Autodesk Inventor part; units mm, degrees
(part 2 of 2)
sketch "Esquisse17" plane through (0, 1.2, 0) normal (0, 1, 0) x (1, 0, 0)
  line L0 (-1.4817, 5.2601) -> (-1.4817, 7.5121) construction
  line L1 (-1.4817, 7.5121) -> (-0.4817, 7.5121) construction
  line L2 (-0.4817, 7.5121) -> (-0.4817, 5.2601) construction
  line L3 (-0.4817, 5.2601) -> (-1.4817, 5.2601) construction
  line L4 (-1.4819, 10.1681) -> (-1.4819, 12.4202) construction
  line L5 (-1.4819, 12.4202) -> (-0.4819, 12.4202) construction
  line L6 (-0.4819, 12.4202) -> (-0.4819, 10.1681) construction
  line L7 (-0.4819, 10.1681) -> (-1.4819, 10.1681) construction
  line L8 (-1.5006, 15.4095) -> (-1.5006, 17.6616) construction
  line L9 (-1.5006, 17.6616) -> (-0.5006, 17.6616) construction
  line L10 (-0.5006, 17.6616) -> (-0.5006, 15.4095) construction
  line L11 (-0.5006, 15.4095) -> (-1.5006, 15.4095) construction
  line L12 (-4.5935, 7.6677) -> (-4.5935, 9.9198) construction
  line L13 (-4.5935, 9.9198) -> (-3.5935, 9.9198) construction
  line L14 (-3.5935, 9.9198) -> (-3.5935, 7.6677) construction
  line L15 (-3.5935, 7.6677) -> (-4.5935, 7.6677) construction
  line L16 (-3.5936, 12.8721) -> (-4.5936, 12.8721) construction
  line L17 (-4.5936, 12.8721) -> (-4.5936, 15.1241) construction
  line L18 (-4.5936, 15.1241) -> (-3.5936, 15.1241) construction
  line L19 (-3.5936, 15.1241) -> (-3.5936, 12.8721) construction
  line L20 (-3.6123, 18.0765) -> (-4.6123, 18.0765) construction
  line L21 (-4.6123, 18.0765) -> (-4.6123, 20.3285) construction
  line L22 (-4.6123, 20.3285) -> (-3.6123, 20.3285) construction
  line L23 (-3.6123, 20.3285) -> (-3.6123, 18.0765) construction
  line L24 (-1.4817, 6.0867) -> (-0.4817, 5.7423)
  line L25 (-0.4817, 5.7423) -> (-0.4817, 5.5988)
  line L26 (-0.4817, 5.5988) -> (-1.4817, 5.2544)
  line L27 (-1.4817, 5.2544) -> (-1.4817, 5.3971)
  line L28 (-1.4817, 5.3971) -> (-0.6511, 5.6742)
  line L29 (-0.6511, 5.6742) -> (-1.4817, 5.9513)
  line L30 (-1.4817, 5.9513) -> (-1.4817, 6.0867)
  line L31 (-0.4817, 6.5308) -> (-0.4817, 6.1434)
  line L32 (-0.4817, 6.1434) -> (-0.5838, 6.1434)
  line L33 (-0.5838, 6.1434) -> (-0.5838, 6.2706)
  line L34 (-0.5838, 6.2706) -> (-1.3796, 6.2706)
  line L35 (-1.3796, 6.2706) -> (-1.3796, 6.1434)
  line L36 (-1.3796, 6.1434) -> (-1.4817, 6.1434)
  line L37 (-1.4817, 6.1434) -> (-1.4817, 6.5308)
  line L38 (-1.4817, 6.5308) -> (-1.3796, 6.5308)
  line L39 (-1.3796, 6.5308) -> (-1.3796, 6.4035)
  line L40 (-1.3796, 6.4035) -> (-0.5838, 6.4035)
  line L41 (-0.5838, 6.4035) -> (-0.5838, 6.5308)
  line L42 (-0.5838, 6.5308) -> (-0.4817, 6.5308)
  line L43 (-0.4817, 7.4108) -> (-0.4817, 7.2617)
  line L44 (-0.4817, 7.2617) -> (-1.344, 6.8193)
  line L45 (-1.344, 6.8193) -> (-0.4817, 6.8193)
  line L46 (-0.4817, 6.8193) -> (-0.4817, 6.6953)
  line L47 (-0.4817, 6.6953) -> (-1.4817, 6.6953)
  line L48 (-1.4817, 6.6953) -> (-1.4817, 6.8841)
  line L49 (-1.4817, 6.8841) -> (-0.69, 7.2868)
  line L50 (-0.69, 7.2868) -> (-1.4817, 7.2868)
  line L51 (-1.4817, 7.2868) -> (-1.4817, 7.4108)
  line L52 (-1.4817, 7.4108) -> (-0.4817, 7.4108)
  spline S0 degree 2 poles (-4.4776, 8.0105) (-4.4776, 7.9741) (-4.4598, 7.9019) (-4.446, 7.8671) knots 0 0 0 1 2 2 2
  spline S1 degree 2 poles (-4.446, 7.8671) (-4.4322, 7.8347) (-4.403, 7.7869) (-4.3901, 7.7682) knots 0 0 0 1 2 2 2
  line L53 (-4.3901, 7.7682) -> (-4.3901, 7.7601)
  line L54 (-4.3901, 7.7601) -> (-4.5319, 7.7601)
  spline S2 degree 2 poles (-4.5319, 7.7601) (-4.5554, 7.8039) (-4.5935, 7.9538) (-4.5935, 8.0211) knots 0 0 0 1 2 2 2
  spline S3 degree 2 poles (-4.5935, 8.0211) (-4.5935, 8.0891) (-4.5659, 8.1904) (-4.5368, 8.2318) knots 0 0 0 1 2 2 2
  spline S4 degree 2 poles (-4.5368, 8.2318) (-4.5052, 8.2755) (-4.4136, 8.3209) (-4.352, 8.3209) knots 0 0 0 1 2 2 2
  spline S5 degree 2 poles (-4.352, 8.3209) (-4.2693, 8.3209) (-4.1445, 8.2123) (-4.1283, 8.1361) knots 0 0 0 1 2 2 2
  line L55 (-4.1283, 8.1361) -> (-4.1186, 8.1361)
  spline S6 degree 2 poles (-4.1186, 8.1361) (-4.1121, 8.1677) (-4.083, 8.2399) (-4.0538, 8.2706) knots 0 0 0 1 2 2 2
  spline S7 degree 2 poles (-4.0538, 8.2706) (-4.0254, 8.3014) (-3.9347, 8.3403) (-3.869, 8.3403) knots 0 0 0 1 2 2 2
  spline S8 degree 2 poles (-3.869, 8.3403) (-3.8018, 8.3403) (-3.6875, 8.2941) (-3.6437, 8.252) knots 0 0 0 1 2 2 2
  spline S9 degree 2 poles (-3.6437, 8.252) (-3.5983, 8.2082) (-3.5513, 8.0843) (-3.5513, 8.0057) knots 0 0 0 1 2 2 2
  spline S10 degree 2 poles (-3.5513, 8.0057) (-3.5513, 7.9303) (-3.5878, 7.7828) (-3.6129, 7.7326) knots 0 0 0 1 2 2 2
  line L56 (-3.6129, 7.7326) -> (-3.7547, 7.7326)
  line L57 (-3.7547, 7.7326) -> (-3.7547, 7.7423)
  spline S11 degree 2 poles (-3.7547, 7.7423) (-3.724, 7.7844) (-3.6672, 7.9271) (-3.6672, 7.9976) knots 0 0 0 1 2 2 2
  spline S12 degree 2 poles (-3.6672, 7.9976) (-3.6672, 8.0389) (-3.6932, 8.1215) (-3.7231, 8.1491) knots 0 0 0 1 2 2 2
  spline S13 degree 2 poles (-3.7231, 8.1491) (-3.7531, 8.1758) (-3.8244, 8.2042) (-3.8787, 8.2042) knots 0 0 0 1 2 2 2
  spline S14 degree 2 poles (-3.8787, 8.2042) (-3.933, 8.2042) (-4.0035, 8.1726) (-4.0238, 8.1442) knots 0 0 0 1 2 2 2
  spline S15 degree 2 poles (-4.0238, 8.1442) (-4.0441, 8.1159) (-4.0594, 8.0389) (-4.0594, 7.9935) knots 0 0 0 1 2 2 2
  line L58 (-4.0594, 7.9935) -> (-4.0594, 7.9368)
  line L59 (-4.0594, 7.9368) -> (-4.1705, 7.9368)
  line L60 (-4.1705, 7.9368) -> (-4.1705, 7.9813)
  spline S16 degree 2 poles (-4.1705, 7.9813) (-4.1705, 8.0713) (-4.2564, 8.1847) (-4.3382, 8.1847) knots 0 0 0 1 2 2 2
  spline S17 degree 2 poles (-4.3382, 8.1847) (-4.3763, 8.1847) (-4.4306, 8.1556) (-4.4468, 8.1321) knots 0 0 0 1 2 2 2
  spline S18 degree 2 poles (-4.4468, 8.1321) (-4.4638, 8.107) (-4.4776, 8.0454) (-4.4776, 8.0105) knots 0 0 0 1 2 2 2
  line L61 (-4.5724, 9.2447) -> (-3.5724, 8.9003)
  line L62 (-3.5724, 8.9003) -> (-3.5724, 8.7569)
  line L63 (-3.5724, 8.7569) -> (-4.5724, 8.4125)
  line L64 (-4.5724, 8.4125) -> (-4.5724, 8.5551)
  line L65 (-4.5724, 8.5551) -> (-3.7418, 8.8322)
  line L66 (-3.7418, 8.8322) -> (-4.5724, 9.1094)
  line L67 (-4.5724, 9.1094) -> (-4.5724, 9.2447)
  spline S19 degree 2 poles (-3.9476, 9.9473) (-3.758, 9.9473) (-3.5513, 9.765) (-3.5513, 9.6126) knots 0 0 0 1 2 2 2
  spline S20 degree 2 poles (-3.5513, 9.6126) (-3.5513, 9.4562) (-3.7645, 9.2771) (-3.9476, 9.2771) knots 0 0 0 1 2 2 2
  spline S21 degree 2 poles (-3.9476, 9.2771) (-4.1356, 9.2771) (-4.3439, 9.4619) (-4.3439, 9.6126) knots 0 0 0 1 2 2 2
  spline S22 degree 2 poles (-4.3439, 9.6126) (-4.3439, 9.765) (-4.1364, 9.9473) (-3.9476, 9.9473) knots 0 0 0 1 2 2 2
  spline S23 degree 2 poles (-3.9476, 9.8168) (-4.0935, 9.8168) (-4.2353, 9.7107) (-4.2353, 9.6126) knots 0 0 0 1 2 2 2
  spline S24 degree 2 poles (-4.2353, 9.6126) (-4.2353, 9.5146) (-4.0935, 9.4076) (-3.9476, 9.4076) knots 0 0 0 1 2 2 2
  spline S25 degree 2 poles (-3.9476, 9.4076) (-3.8058, 9.4076) (-3.6599, 9.5146) (-3.6599, 9.6126) knots 0 0 0 1 2 2 2
  spline S26 degree 2 poles (-3.6599, 9.6126) (-3.6599, 9.7099) (-3.8034, 9.8168) (-3.9476, 9.8168) knots 0 0 0 1 2 2 2
  spline S27 degree 2 poles (-3.558, 13.2522) (-3.558, 13.1436) (-3.6034, 12.9912) (-3.6358, 12.924) knots 0 0 0 1 2 2 2
  line L68 (-3.6358, 12.924) -> (-3.8027, 12.924)
  line L69 (-3.8027, 12.924) -> (-3.8027, 12.9337)
  spline S28 degree 2 poles (-3.8027, 12.9337) (-3.7411, 12.9993) (-3.6731, 13.1655) (-3.6731, 13.2424) knots 0 0 0 1 2 2 2
  spline S29 degree 2 poles (-3.6731, 13.2424) (-3.6731, 13.3527) (-3.7646, 13.4653) (-3.84, 13.4653) knots 0 0 0 1 2 2 2
  spline S30 degree 2 poles (-3.84, 13.4653) (-3.9, 13.4653) (-3.9745, 13.4061) (-3.9932, 13.3421) knots 0 0 0 1 2 2 2
  spline S31 degree 2 poles (-3.9932, 13.3421) (-4.0061, 13.2959) (-4.024, 13.2189) (-4.0385, 13.1614) knots 0 0 0 1 2 2 2
  spline S32 degree 2 poles (-4.0385, 13.1614) (-4.0523, 13.1095) (-4.0936, 13.0277) (-4.1269, 12.9961) knots 0 0 0 1 2 2 2
  spline S33 degree 2 poles (-4.1269, 12.9961) (-4.1601, 12.9653) (-4.2492, 12.9313) (-4.3076, 12.9313) knots 0 0 0 1 2 2 2
  spline S34 degree 2 poles (-4.3076, 12.9313) (-4.4291, 12.9313) (-4.5936, 13.1209) (-4.5936, 13.2676) knots 0 0 0 1 2 2 2
  spline S35 degree 2 poles (-4.5936, 13.2676) (-4.5936, 13.3518) (-4.5604, 13.501) (-4.5288, 13.565) knots 0 0 0 1 2 2 2
  line L70 (-4.5288, 13.565) -> (-4.37, 13.565)
  line L71 (-4.37, 13.565) -> (-4.37, 13.5553)
  spline S36 degree 2 poles (-4.37, 13.5553) (-4.4137, 13.5074) (-4.4786, 13.3583) (-4.4786, 13.2765) knots 0 0 0 1 2 2 2
  spline S37 degree 2 poles (-4.4786, 13.2765) (-4.4786, 13.1841) (-4.3919, 13.0698) (-4.3214, 13.0698) knots 0 0 0 1 2 2 2
  spline S38 degree 2 poles (-4.3214, 13.0698) (-4.2582, 13.0698) (-4.1828, 13.1371) (-4.1658, 13.2003) knots 0 0 0 1 2 2 2
  spline S39 degree 2 poles (-4.1658, 13.2003) (-4.1544, 13.2424) (-4.1252, 13.3648) (-4.1131, 13.4053) knots 0 0 0 1 2 2 2
  spline S40 degree 2 poles (-4.1131, 13.4053) (-4.0815, 13.5082) (-3.9543, 13.6039) (-3.8611, 13.6039) knots 0 0 0 1 2 2 2
  spline S41 degree 2 poles (-3.8611, 13.6039) (-3.8019, 13.6039) (-3.6885, 13.5561) (-3.6488, 13.5131) knots 0 0 0 1 2 2 2
  spline S42 degree 2 poles (-3.6488, 13.5131) (-3.605, 13.4653) (-3.558, 13.3437) (-3.558, 13.2522) knots 0 0 0 1 2 2 2
  spline S43 degree 2 poles (-3.558, 14.1298) (-3.558, 14.0326) (-3.6236, 13.8681) (-3.6893, 13.8081) knots 0 0 0 1 2 2 2
  spline S44 degree 2 poles (-3.6893, 13.8081) (-3.7541, 13.7481) (-3.9486, 13.6825) (-4.075, 13.6825) knots 0 0 0 1 2 2 2
  spline S45 degree 2 poles (-4.075, 13.6825) (-4.2006, 13.6825) (-4.387, 13.7465) (-4.4559, 13.8073) knots 0 0 0 1 2 2 2
  spline S46 degree 2 poles (-4.4559, 13.8073) (-4.5231, 13.8672) (-4.5936, 14.0309) (-4.5936, 14.1322) knots 0 0 0 1 2 2 2
  spline S47 degree 2 poles (-4.5936, 14.1322) (-4.5936, 14.1825) (-4.5791, 14.2708) (-4.5677, 14.3081) knots 0 0 0 1 2 2 2
  spline S48 degree 2 poles (-4.5677, 14.3081) (-4.5572, 14.3405) (-4.5272, 14.4078) (-4.5094, 14.441) knots 0 0 0 1 2 2 2
  line L72 (-4.5094, 14.441) -> (-4.3489, 14.441)
  line L73 (-4.3489, 14.441) -> (-4.3489, 14.4305)
  spline S49 degree 2 poles (-4.3489, 14.4305) (-4.3651, 14.4126) (-4.4105, 14.3575) (-4.4324, 14.3178) knots 0 0 0 1 2 2 2
  spline S50 degree 2 poles (-4.4324, 14.3178) (-4.4535, 14.2797) (-4.4802, 14.1898) (-4.4802, 14.1314) knots 0 0 0 1 2 2 2
  spline S51 degree 2 poles (-4.4802, 14.1314) (-4.4802, 14.0674) (-4.4275, 13.9531) (-4.3773, 13.9102) knots 0 0 0 1 2 2 2
  spline S52 degree 2 poles (-4.3773, 13.9102) (-4.3262, 13.8681) (-4.1714, 13.8211) (-4.075, 13.8211) knots 0 0 0 1 2 2 2
  spline S53 degree 2 poles (-4.075, 13.8211) (-3.9721, 13.8211) (-3.8238, 13.8705) (-3.7727, 13.9134) knots 0 0 0 1 2 2 2
  spline S54 degree 2 poles (-3.7727, 13.9134) (-3.7233, 13.9556) (-3.6731, 14.0682) (-3.6731, 14.1314) knots 0 0 0 1 2 2 2
  spline S55 degree 2 poles (-3.6731, 14.1314) (-3.6731, 14.189) (-3.7014, 14.287) (-3.7225, 14.3251) knots 0 0 0 1 2 2 2
  spline S56 degree 2 poles (-3.7225, 14.3251) (-3.7436, 14.3616) (-3.7873, 14.4159) (-3.8027, 14.4313) knots 0 0 0 1 2 2 2
  line L74 (-3.8027, 14.4313) -> (-3.8027, 14.441)
  line L75 (-3.8027, 14.441) -> (-3.6439, 14.441)
  spline S57 degree 2 poles (-3.6439, 14.441) (-3.6285, 14.4078) (-3.6001, 14.3494) (-3.5872, 14.3081) knots 0 0 0 1 2 2 2
  spline S58 degree 2 poles (-3.5872, 14.3081) (-3.5726, 14.2643) (-3.558, 14.1898) (-3.558, 14.1298) knots 0 0 0 1 2 2 2
  line L76 (-3.5758, 15.1444) -> (-3.5758, 14.565)
  line L77 (-3.5758, 14.565) -> (-4.5758, 14.565)
  line L78 (-4.5758, 14.565) -> (-4.5758, 14.6979)
  line L79 (-4.5758, 14.6979) -> (-3.6941, 14.6979)
  line L80 (-3.6941, 14.6979) -> (-3.6941, 15.1444)
  line L81 (-3.6941, 15.1444) -> (-3.5758, 15.1444)
  line L82 (-3.6123, 18.5262) -> (-3.6123, 18.1389)
  line L83 (-3.6123, 18.1389) -> (-3.7144, 18.1389)
  line L84 (-3.7144, 18.1389) -> (-3.7144, 18.2661)
  line L85 (-3.7144, 18.2661) -> (-4.5102, 18.2661)
  line L86 (-4.5102, 18.2661) -> (-4.5102, 18.1389)
  line L87 (-4.5102, 18.1389) -> (-4.6123, 18.1389)
  line L88 (-4.6123, 18.1389) -> (-4.6123, 18.5262)
  line L89 (-4.6123, 18.5262) -> (-4.5102, 18.5262)
  line L90 (-4.5102, 18.5262) -> (-4.5102, 18.399)
  line L91 (-4.5102, 18.399) -> (-3.7144, 18.399)
  line L92 (-3.7144, 18.399) -> (-3.7144, 18.5262)
  line L93 (-3.7144, 18.5262) -> (-3.6123, 18.5262)
  line L94 (-3.6123, 19.4063) -> (-3.6123, 19.2572)
  line L95 (-3.6123, 19.2572) -> (-4.4746, 18.8147)
  line L96 (-4.4746, 18.8147) -> (-3.6123, 18.8147)
  line L97 (-3.6123, 18.8147) -> (-3.6123, 18.6907)
  line L98 (-3.6123, 18.6907) -> (-4.6123, 18.6907)
  line L99 (-4.6123, 18.6907) -> (-4.6123, 18.8796)
  line L100 (-4.6123, 18.8796) -> (-3.8206, 19.2823)
  line L101 (-3.8206, 19.2823) -> (-4.6123, 19.2823)
  line L102 (-4.6123, 19.2823) -> (-4.6123, 19.4063)
  line L103 (-4.6123, 19.4063) -> (-3.6123, 19.4063)
  line L104 (-3.6123, 19.8423) -> (-4.494, 19.8423)
  line L105 (-4.494, 19.8423) -> (-4.494, 19.5068)
  line L106 (-4.494, 19.5068) -> (-4.6123, 19.5068)
  line L107 (-4.6123, 19.5068) -> (-4.6123, 20.3107)
  line L108 (-4.6123, 20.3107) -> (-4.494, 20.3107)
  line L109 (-4.494, 20.3107) -> (-4.494, 19.9752)
  line L110 (-4.494, 19.9752) -> (-3.6123, 19.9752)
  line L111 (-3.6123, 19.9752) -> (-3.6123, 19.8423)
  spline S59 degree 2 poles (-0.4649, 15.7896) (-0.4649, 15.681) (-0.5103, 15.5287) (-0.5427, 15.4614) knots 0 0 0 1 2 2 2
  line L112 (-0.5427, 15.4614) -> (-0.7096, 15.4614)
  line L113 (-0.7096, 15.4614) -> (-0.7096, 15.4711)
  spline S60 degree 2 poles (-0.7096, 15.4711) (-0.648, 15.5368) (-0.58, 15.7029) (-0.58, 15.7799) knots 0 0 0 1 2 2 2
  spline S61 degree 2 poles (-0.58, 15.7799) (-0.58, 15.8901) (-0.6715, 16.0027) (-0.7469, 16.0027) knots 0 0 0 1 2 2 2
  spline S62 degree 2 poles (-0.7469, 16.0027) (-0.8069, 16.0027) (-0.8814, 15.9436) (-0.9001, 15.8796) knots 0 0 0 1 2 2 2
  spline S63 degree 2 poles (-0.9001, 15.8796) (-0.913, 15.8334) (-0.9309, 15.7564) (-0.9455, 15.6989) knots 0 0 0 1 2 2 2
  spline S64 degree 2 poles (-0.9455, 15.6989) (-0.9592, 15.647) (-1.0006, 15.5651) (-1.0338, 15.5335) knots 0 0 0 1 2 2 2
  spline S65 degree 2 poles (-1.0338, 15.5335) (-1.067, 15.5027) (-1.1562, 15.4687) (-1.2145, 15.4687) knots 0 0 0 1 2 2 2
  spline S66 degree 2 poles (-1.2145, 15.4687) (-1.3361, 15.4687) (-1.5006, 15.6583) (-1.5006, 15.805) knots 0 0 0 1 2 2 2
  spline S67 degree 2 poles (-1.5006, 15.805) (-1.5006, 15.8893) (-1.4673, 16.0384) (-1.4357, 16.1024) knots 0 0 0 1 2 2 2
  line L114 (-1.4357, 16.1024) -> (-1.2769, 16.1024)
  line L115 (-1.2769, 16.1024) -> (-1.2769, 16.0927)
  spline S68 degree 2 poles (-1.2769, 16.0927) (-1.3207, 16.0449) (-1.3855, 15.8958) (-1.3855, 15.8139) knots 0 0 0 1 2 2 2
  spline S69 degree 2 poles (-1.3855, 15.8139) (-1.3855, 15.7215) (-1.2988, 15.6073) (-1.2283, 15.6073) knots 0 0 0 1 2 2 2
  spline S70 degree 2 poles (-1.2283, 15.6073) (-1.1651, 15.6073) (-1.0897, 15.6745) (-1.0727, 15.7377) knots 0 0 0 1 2 2 2
  spline S71 degree 2 poles (-1.0727, 15.7377) (-1.0613, 15.7799) (-1.0322, 15.9023) (-1.02, 15.9428) knots 0 0 0 1 2 2 2
  spline S72 degree 2 poles (-1.02, 15.9428) (-0.9884, 16.0457) (-0.8612, 16.1413) (-0.768, 16.1413) knots 0 0 0 1 2 2 2
  spline S73 degree 2 poles (-0.768, 16.1413) (-0.7088, 16.1413) (-0.5954, 16.0935) (-0.5557, 16.0506) knots 0 0 0 1 2 2 2
  spline S74 degree 2 poles (-0.5557, 16.0506) (-0.5119, 16.0027) (-0.4649, 15.8812) (-0.4649, 15.7896) knots 0 0 0 1 2 2 2
  spline S75 degree 2 poles (-0.9819, 17.0651) (-0.845, 17.0651) (-0.6245, 16.9541) (-0.563, 16.8609) knots 0 0 0 1 2 2 2
  spline S76 degree 2 poles (-0.563, 16.8609) (-0.5151, 16.7848) (-0.4827, 16.6283) (-0.4827, 16.5068) knots 0 0 0 1 2 2 2
  line L116 (-0.4827, 16.5068) -> (-0.4827, 16.2766)
  line L117 (-0.4827, 16.2766) -> (-1.4827, 16.2766)
  line L118 (-1.4827, 16.2766) -> (-1.4827, 16.5044)
  spline S77 degree 2 poles (-1.4827, 16.5044) (-1.4827, 16.6454) (-1.4406, 16.8058) (-1.4033, 16.8625) knots 0 0 0 1 2 2 2
  spline S78 degree 2 poles (-1.4033, 16.8625) (-1.3393, 16.959) (-1.1278, 17.0651) (-0.9819, 17.0651) knots 0 0 0 1 2 2 2
  spline S79 degree 2 poles (-0.9835, 16.9266) (-1.0986, 16.9266) (-1.2615, 16.8504) (-1.3077, 16.775) knots 0 0 0 1 2 2 2
  spline S80 degree 2 poles (-1.3077, 16.775) (-1.3393, 16.7215) (-1.3677, 16.6008) (-1.3677, 16.5108) knots 0 0 0 1 2 2 2
  line L119 (-1.3677, 16.5108) -> (-1.3677, 16.4095)
  line L120 (-1.3677, 16.4095) -> (-0.5978, 16.4095)
  line L121 (-0.5978, 16.4095) -> (-0.5978, 16.5108)
  spline S81 degree 2 poles (-0.5978, 16.5108) (-0.5978, 16.5992) (-0.6262, 16.7329) (-0.6643, 16.7872) knots 0 0 0 1 2 2 2
  spline S82 degree 2 poles (-0.6643, 16.7872) (-0.7113, 16.8569) (-0.8668, 16.9266) (-0.9835, 16.9266) knots 0 0 0 1 2 2 2
  line L122 (-0.4827, 17.1016) -> (-1.4827, 17.4387)
  line L123 (-1.4827, 17.4387) -> (-1.4827, 17.6024)
  line L124 (-1.4827, 17.6024) -> (-0.4827, 17.9395)
  line L125 (-0.4827, 17.9395) -> (-0.4827, 17.7993)
  line L126 (-0.4827, 17.7993) -> (-0.7623, 17.7086)
  line L127 (-0.7623, 17.7086) -> (-0.7623, 17.3269)
  line L128 (-0.7623, 17.3269) -> (-0.4827, 17.2361)
  line L129 (-0.4827, 17.2361) -> (-0.4827, 17.1016)
  line L130 (-0.8758, 17.6721) -> (-1.3466, 17.5173)
  line L131 (-1.3466, 17.5173) -> (-0.8758, 17.3634)
  line L132 (-0.8758, 17.3634) -> (-0.8758, 17.6721)
  spline S83 degree 2 poles (-0.4446, 10.6884) (-0.4446, 10.5822) (-0.5094, 10.4064) (-0.5751, 10.3432) knots 0 0 0 1 2 2 2
  spline S84 degree 2 poles (-0.5751, 10.3432) (-0.6415, 10.28) (-0.8376, 10.2127) (-0.9649, 10.2127) knots 0 0 0 1 2 2 2
  spline S85 degree 2 poles (-0.9649, 10.2127) (-1.0856, 10.2127) (-1.2769, 10.2808) (-1.3449, 10.344) knots 0 0 0 1 2 2 2
  spline S86 degree 2 poles (-1.3449, 10.344) (-1.4106, 10.4048) (-1.4819, 10.583) (-1.4819, 10.6892) knots 0 0 0 1 2 2 2
  spline S87 degree 2 poles (-1.4819, 10.6892) (-1.4819, 10.7403) (-1.4673, 10.8326) (-1.4543, 10.8748) knots 0 0 0 1 2 2 2
  spline S88 degree 2 poles (-1.4543, 10.8748) (-1.4446, 10.9088) (-1.4089, 10.9915) (-1.396, 11.0166) knots 0 0 0 1 2 2 2
  line L133 (-1.396, 11.0166) -> (-1.2355, 11.0166)
  line L134 (-1.2355, 11.0166) -> (-1.2355, 11.0052)
  spline S89 degree 2 poles (-1.2355, 11.0052) (-1.2574, 10.9801) (-1.2971, 10.9274) (-1.3198, 10.8788) knots 0 0 0 1 2 2 2
  spline S90 degree 2 poles (-1.3198, 10.8788) (-1.3401, 10.8383) (-1.3668, 10.7338) (-1.3668, 10.6738) knots 0 0 0 1 2 2 2
  spline S91 degree 2 poles (-1.3668, 10.6738) (-1.3668, 10.5296) (-1.1496, 10.3513) (-0.9689, 10.3513) knots 0 0 0 1 2 2 2
  spline S92 degree 2 poles (-0.9689, 10.3513) (-0.8684, 10.3513) (-0.7177, 10.3983) (-0.6658, 10.4428) knots 0 0 0 1 2 2 2
  spline S93 degree 2 poles (-0.6658, 10.4428) (-0.614, 10.4858) (-0.5597, 10.6074) (-0.5597, 10.6835) knots 0 0 0 1 2 2 2
  spline S94 degree 2 poles (-0.5597, 10.6835) (-0.5597, 10.7394) (-0.5759, 10.8513) (-0.5921, 10.8894) knots 0 0 0 1 2 2 2
  line L135 (-0.5921, 10.8894) -> (-0.8506, 10.8894)
  line L136 (-0.8506, 10.8894) -> (-0.8506, 10.6576)
  line L137 (-0.8506, 10.6576) -> (-0.9673, 10.6576)
  line L138 (-0.9673, 10.6576) -> (-0.9673, 11.0206)
  line L139 (-0.9673, 11.0206) -> (-0.5305, 11.0206)
  spline S95 degree 2 poles (-0.5305, 11.0206) (-0.5192, 10.9955) (-0.4843, 10.9096) (-0.4738, 10.8732) knots 0 0 0 1 2 2 2
  spline S96 degree 2 poles (-0.4738, 10.8732) (-0.4592, 10.8237) (-0.4446, 10.7443) (-0.4446, 10.6884) knots 0 0 0 1 2 2 2
  line L140 (-0.464, 11.9031) -> (-0.464, 11.754)
  line L141 (-0.464, 11.754) -> (-1.3263, 11.3116)
  line L142 (-1.3263, 11.3116) -> (-0.464, 11.3116)
  line L143 (-0.464, 11.3116) -> (-0.464, 11.1876)
  line L144 (-0.464, 11.1876) -> (-1.464, 11.1876)
  line L145 (-1.464, 11.1876) -> (-1.464, 11.3764)
  line L146 (-1.464, 11.3764) -> (-0.6723, 11.7792)
  line L147 (-0.6723, 11.7792) -> (-1.464, 11.7792)
  line L148 (-1.464, 11.7792) -> (-1.464, 11.9031)
  line L149 (-1.464, 11.9031) -> (-0.464, 11.9031)
  spline S97 degree 2 poles (-0.9632, 12.8942) (-0.8263, 12.8942) (-0.6059, 12.7832) (-0.5443, 12.69) knots 0 0 0 1 2 2 2
  spline S98 degree 2 poles (-0.5443, 12.69) (-0.4965, 12.6138) (-0.464, 12.4574) (-0.464, 12.3359) knots 0 0 0 1 2 2 2
  line L150 (-0.464, 12.3359) -> (-0.464, 12.1057)
  line L151 (-0.464, 12.1057) -> (-1.464, 12.1057)
  line L152 (-1.464, 12.1057) -> (-1.464, 12.3334)
  spline S99 degree 2 poles (-1.464, 12.3334) (-1.464, 12.4745) (-1.4219, 12.6349) (-1.3846, 12.6916) knots 0 0 0 1 2 2 2
  spline S100 degree 2 poles (-1.3846, 12.6916) (-1.3206, 12.7881) (-1.1091, 12.8942) (-0.9632, 12.8942) knots 0 0 0 1 2 2 2
  spline S101 degree 2 poles (-0.9649, 12.7557) (-1.0799, 12.7557) (-1.2428, 12.6795) (-1.289, 12.6041) knots 0 0 0 1 2 2 2
  spline S102 degree 2 poles (-1.289, 12.6041) (-1.3206, 12.5506) (-1.349, 12.4299) (-1.349, 12.3399) knots 0 0 0 1 2 2 2
  line L153 (-1.349, 12.3399) -> (-1.349, 12.2386)
  line L154 (-1.349, 12.2386) -> (-0.5791, 12.2386)
  line L155 (-0.5791, 12.2386) -> (-0.5791, 12.3399)
  spline S103 degree 2 poles (-0.5791, 12.3399) (-0.5791, 12.4283) (-0.6075, 12.562) (-0.6456, 12.6163) knots 0 0 0 1 2 2 2
  spline S104 degree 2 poles (-0.6456, 12.6163) (-0.6926, 12.686) (-0.8482, 12.7557) (-0.9649, 12.7557) knots 0 0 0 1 2 2 2
  point P0 (0, 0)
  constraints: 12 other
extrude "Extrusion21" cut sketch "Esquisse17" against normal blind 0.01
sketch "Esquisse18" plane through (0, 1.2, 0) normal (0, 1, 0) x (1, 0, 0)
  line L0 (-7.89, 11.95) -> (-9.89, 11.95) projected
  line L1 (-9.89, 11.95) -> (-9.89, 13.45) projected
  line L2 (-7.89, 11.95) -> (-9.89, 11.95)
  line L3 (-9.89, 11.95) -> (-9.89, 13.45)
  line L4 (-9.89, 13.45) -> (-7.89, 13.45)
  line L5 (-7.89, 13.45) -> (-7.89, 11.95)
  line L6 (-8.19, 13.15) -> (-9.59, 13.15)
  line L7 (-9.59, 13.15) -> (-9.59, 12.25)
  line L8 (-9.59, 12.25) -> (-8.19, 12.25)
  line L9 (-8.19, 12.25) -> (-8.19, 13.15)
  point P0 (0, 0)
  dimension "d179" = 0.3
  constraints: 16 end point, 4 parallel, 2 perpendicular, 1 horizontal, 3 other
  measures "d179" distance between parallel lines of L4 L6
extrude "Extrusion22" cut sketch "Esquisse18" along normal blind 0.25 contours L9 L8 L7 L6
equation "\"d65\" = d64"
equation "\"d68\" = d67"
equation "\"d71\" = d70"
